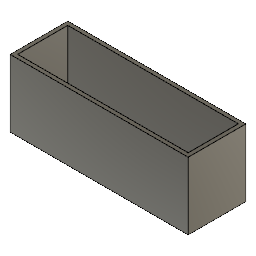
First Test Fit v8 (Autodesk Fusion 360 archive; units mm, degrees)
design "nerf based hopper housing bottom"
Autodesk Fusion 360 part; units mm, degrees
box "BoxPrimitive1" add length 76.2 width 234.95 height 88.9 placed x (0, -1, 0) y (1, 0, 0) z (0, 0, 1) at (0, 0, 0)
shell "Shell1" thickness 5.08 removed faces 1 at (78.3167, -25.4, 88.9)
sketch "flywheel axle" plane through (5.08, 0, 0) normal (1, 0, 0) x (0, 1, 0)
  line L0 (-5.08, 5.08) -> (-5.08, 88.9)
  line L1 (-5.08, 88.9) -> (-71.12, 88.9)
  line L2 (-71.12, 88.9) -> (-71.12, 5.08)
  line L3 (-71.12, 5.08) -> (-5.08, 5.08)
  line L4 (-38.1, 88.9) -> (-38.1, 5.08) construction
  line L5 (-71.12, 46.99) -> (-5.08, 46.99) construction
  circle A0 centre (-38.1, 46.99) radius 3.1
  point P0 (-38.1, 46.99)
  dimension "d10" = 6.2
  constraint midpoint L1 L4.start
  constraint midpoint L3 L4.end
  constraint midpoint L2 L5.start
  constraint midpoint L0 L5.end
  constraint midpoint L4 P0
  constraint coincident P0 A0.centre
  measures "d10" diameter of A0
extrude "Extrude1" add sketch "flywheel axle" along normal blind 228.6 contours A0
sketch "tube slot" plane through (0, 0, 0) normal (0, 1, 0) x (-1, 0, 0)
  line L0 (-234.95, 88.9) -> (-234.95, 0)
  line L1 (-234.95, 0) -> (0, 0)
  line L2 (0, 0) -> (0, 88.9)
  line L3 (0, 88.9) -> (-234.95, 88.9)
  line L4 (-233.68, 11.3178) -> (-1.905, 11.3178)
  line L5 (-1.905, 11.3178) -> (-1.905, 5.08)
  line L6 (-1.905, 5.08) -> (-233.68, 5.08)
  line L7 (-233.68, 5.08) -> (-233.68, 11.3178)
  dimension "d11" = 231.775
  dimension "d13" = 6.2378
  dimension "d14" = 1.27
  dimension "d15" = 5.08
  constraint horizontal L4
  constraint vertical L5
  constraint horizontal L6
  constraint vertical L7
  measures "d11" distance of L4.start L4.end
  measures "d13" distance of L4.end L5.end
  measures "d14" distance of L0 L7
  measures "d15" distance of L1 L6
extrude "Extrude2" cut sketch "tube slot" against normal blind 12.7 contours L4 L5 L6 L7
named bodies: "bottom hopper"

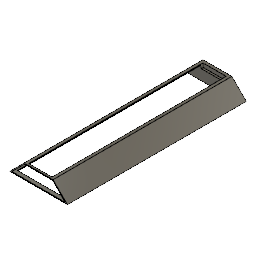
design "nerf based hopper housing V2"
Autodesk Fusion 360 part; units mm, degrees
sketch "top hopper side" plane through (0, 0, 0) normal (0, 1, 0) x (1, 0, 0)
  line L0 (-76.2, 0) -> (0, 0)
  line L1 (0, 0) -> (-19.05, -19.05)
  line L2 (-19.05, -19.05) -> (-57.15, -19.05)
  line L3 (-57.15, -19.05) -> (-76.2, 0)
  dimension "d12" = 76.2
  dimension "d13" = 38.1
  dimension "d14" = 45
  constraint horizontal L0
  constraint parallel L0 L2
  constraint perpendicular L1 L3
  constraint coincident L0.end L1.start
  measures "d12" distance of L0.start L0.end
  measures "d13" distance of L1.end L2.end
  measures "d14" angle of L0 L1
extrude "Extrude3" add sketch "top hopper side" along normal blind 234.95
sketch "side cutout" plane through (0, 0, 0) normal (0, -1, 0) x (1, 0, 0)
  line L0 (-19.05, 19.05) -> (-57.15, 19.05)
  line L1 (-57.15, 19.05) -> (-76.2, 0)
  line L2 (-76.2, 0) -> (0, 0)
  line L3 (0, 0) -> (-19.05, 19.05)
  line L4 (-76.2, 0) -> (-57.15, 19.05)
  line L5 (-19.05, 19.05) -> (0, 0)
  line L6 (-76.2, 0) -> (0, 0)
  line L7 (-57.15, 19.05) -> (-19.05, 19.05)
  line L8 (-73.1339, 1.27) -> (-3.0661, 1.27)
  line L9 (-19.5761, 17.78) -> (-3.0661, 1.27)
  line L10 (-56.6239, 17.78) -> (-19.5761, 17.78)
  line L11 (-73.1339, 1.27) -> (-56.6239, 17.78)
  dimension "d17" = 1.27
  constraint coincident L1.end L2.start
  constraint coincident L0.end L1.start
  constraint coincident L0.start L3.end
  constraint coincident L2.end L3.start
extrude "Extrude4" cut sketch "side cutout" against normal blind 228.6 contours L8 L9 L10 L11
sketch "bottom cutout" plane through (0, 0, 0) normal (0, 0, -1) x (1, 0, 0)
  line L0 (0, 0) -> (-76.2, 0)
  line L1 (-76.2, 0) -> (-76.2, -234.95)
  line L2 (-76.2, -234.95) -> (0, -234.95)
  line L3 (0, -234.95) -> (0, 0)
  line L4 (-5.08, -5.08) -> (-70.7474, -5.08)
  line L5 (-70.7474, -5.08) -> (-70.7474, -228.6)
  line L6 (-5.08, -228.6) -> (-5.08, -5.08)
  line L7 (-5.08, -228.6) -> (-70.7474, -228.6)
  dimension "d20" = 223.52
  dimension "d21" = 65.6674
  dimension "d22" = 5.08
  dimension "d23" = 5.08
  constraint horizontal L4
  constraint vertical L5
  constraint vertical L6
  constraint perpendicular L5 L7
  measures "d20" distance of L4.start L6.start
  measures "d21" distance of L5.end L6.start
  measures "d22" distance of L3 L6
  measures "d23" distance of L0 L4
extrude "Extrude5" cut sketch "bottom cutout" against normal blind 2.54 contours L4 L5 L6 L7
sketch "top cutout" plane through (0, 0, 19.05) normal (0, 0, 1) x (-1, 0, 0)
  line L0 (57.15, 0) -> (19.05, 0)
  line L1 (19.05, 0) -> (19.05, -234.95)
  line L2 (19.05, -234.95) -> (57.15, -234.95)
  line L3 (57.15, -234.95) -> (57.15, 0)
  line L4 (53.34, -2.54) -> (22.86, -2.54)
  line L5 (22.86, -2.54) -> (22.86, -231.14)
  line L6 (22.86, -231.14) -> (53.34, -231.14)
  line L7 (53.34, -231.14) -> (53.34, -2.54)
  dimension "d26" = 228.6
  dimension "d27" = 30.48
  dimension "d28" = 3.81
  dimension "d29" = 2.54
  constraint horizontal L4
  constraint vertical L5
  constraint horizontal L6
  constraint vertical L7
  measures "d26" distance of L4.start L6.end
  measures "d27" distance of L5.end L6.end
  measures "d28" distance of L3 L7
  measures "d29" distance of L0 L4
extrude "Extrude6" cut sketch "top cutout" against normal blind 5.08 contours L4 L5 L6 L7
named bodies: "top hopper"

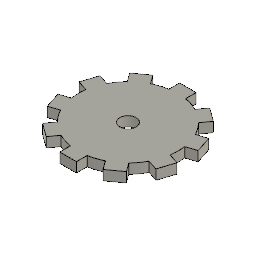
design "Flywheel idea"
Autodesk Fusion 360 part; units mm, degrees
sketch "wheel" plane through (0, 0, 0) normal (0, 0, 1) x (1, 0, 0)
  circle A0 centre (0, 0) radius 19.05
  line L0 (-3.1964, 18.7799) -> (-3.1964, 22.86)
  line L1 (-3.1964, 22.86) -> (3.1964, 22.86)
  line L2 (3.1964, 22.86) -> (3.1964, 18.7799)
  line L3 (-13.6245, 13.3144) -> (-16.0227, 16.6153)
  line L4 (-16.0227, 16.6153) -> (-10.8508, 20.3729)
  line L5 (-10.8508, 20.3729) -> (-8.4526, 17.0721)
  line L6 (-18.8485, 2.7633) -> (-22.7289, 4.0241)
  line L7 (-22.7289, 4.0241) -> (-20.7534, 10.1041)
  line L8 (-20.7534, 10.1041) -> (-16.873, 8.8433)
  line L9 (-16.873, -8.8433) -> (-20.7534, -10.1041)
  line L10 (-20.7534, -10.1041) -> (-22.7289, -4.0241)
  line L11 (-22.7289, -4.0241) -> (-18.8485, -2.7633)
  line L12 (-8.4526, -17.0721) -> (-10.8508, -20.373)
  line L13 (-10.8508, -20.373) -> (-16.0227, -16.6153)
  line L14 (-16.0227, -16.6153) -> (-13.6245, -13.3145)
  line L15 (3.1964, -18.7799) -> (3.1964, -22.86)
  line L16 (3.1964, -22.86) -> (-3.1964, -22.86)
  line L17 (-3.1964, -22.86) -> (-3.1964, -18.7799)
  line L18 (13.6245, -13.3144) -> (16.0227, -16.6153)
  line L19 (16.0227, -16.6153) -> (10.8508, -20.3729)
  line L20 (10.8508, -20.3729) -> (8.4526, -17.0721)
  line L21 (18.8485, -2.7633) -> (22.7289, -4.0241)
  line L22 (22.7289, -4.0241) -> (20.7534, -10.1041)
  line L23 (20.7534, -10.1041) -> (16.873, -8.8433)
  line L24 (16.873, 8.8433) -> (20.7534, 10.1041)
  line L25 (20.7534, 10.1041) -> (22.7289, 4.0241)
  line L26 (22.7289, 4.0241) -> (18.8485, 2.7633)
  line L27 (8.4526, 17.0721) -> (10.8508, 20.373)
  line L28 (10.8508, 20.373) -> (16.0227, 16.6153)
  line L29 (16.0227, 16.6153) -> (13.6245, 13.3145)
  dimension "d1" = 38.1
  dimension "d2" = 6.3929
  dimension "d3" = 4.0801
  dimension "d5" = 360
  constraint coincident A0.centre origin
  constraint coincident A0 L0.start
  constraint vertical L0
  constraint perpendicular L0 L1
  constraint coincident A0 L2.end
  constraint perpendicular L1 L2
  constraint equal L0 L2
  measures "d1" diameter of A0
  measures "d2" distance of L0.end L1.end
  measures "d3" distance of L1.end L2.end
extrude "Extrude1" add sketch "wheel" along normal blind 3.81
sketch "hole punch" plane through (0, 0, 3.81) normal (0, 0, 1) x (-1, 0, 0)
  arc A0 (-8.4526, -17.0721) -> (-3.1964, -18.7799) centre (0, 0) ccw
  line L0 (-3.1964, -18.7799) -> (-3.1964, -22.86)
  line L1 (-3.1964, -22.86) -> (3.1964, -22.86)
  line L2 (3.1964, -22.86) -> (3.1964, -18.7799)
  arc A1 (3.1964, -18.7799) -> (8.4526, -17.0721) centre (0, 0) ccw
  line L3 (8.4526, -17.0721) -> (10.8508, -20.3729)
  line L4 (10.8508, -20.3729) -> (16.0227, -16.6153)
  line L5 (16.0227, -16.6153) -> (13.6245, -13.3144)
  arc A2 (13.6245, -13.3144) -> (16.873, -8.8433) centre (0, 0) ccw
  line L6 (16.873, -8.8433) -> (20.7534, -10.1041)
  line L7 (20.7534, -10.1041) -> (22.7289, -4.0241)
  line L8 (22.7289, -4.0241) -> (18.8485, -2.7633)
  arc A3 (18.8485, -2.7633) -> (18.8485, 2.7633) centre (0, 0) ccw
  line L9 (18.8485, 2.7633) -> (22.7289, 4.0241)
  line L10 (22.7289, 4.0241) -> (20.7534, 10.1041)
  line L11 (20.7534, 10.1041) -> (16.873, 8.8433)
  arc A4 (16.873, 8.8433) -> (13.6245, 13.3145) centre (0, 0) ccw
  line L12 (13.6245, 13.3145) -> (16.0227, 16.6153)
  line L13 (16.0227, 16.6153) -> (10.8508, 20.373)
  line L14 (10.8508, 20.373) -> (8.4526, 17.0721)
  arc A5 (8.4526, 17.0721) -> (3.1964, 18.7799) centre (0, 0) ccw
  line L15 (3.1964, 18.7799) -> (3.1964, 22.86)
  line L16 (3.1964, 22.86) -> (-3.1964, 22.86)
  line L17 (-3.1964, 22.86) -> (-3.1964, 18.7799)
  arc A6 (-3.1964, 18.7799) -> (-8.4526, 17.0721) centre (0, 0) ccw
  line L18 (-8.4526, 17.0721) -> (-10.8508, 20.3729)
  line L19 (-10.8508, 20.3729) -> (-16.0227, 16.6153)
  line L20 (-16.0227, 16.6153) -> (-13.6245, 13.3144)
  arc A7 (-13.6245, 13.3144) -> (-16.873, 8.8433) centre (0, 0) ccw
  line L21 (-16.873, 8.8433) -> (-20.7534, 10.1041)
  line L22 (-20.7534, 10.1041) -> (-22.7289, 4.0241)
  line L23 (-22.7289, 4.0241) -> (-18.8485, 2.7633)
  arc A8 (-18.8485, 2.7633) -> (-18.8485, -2.7633) centre (0, 0) ccw
  line L24 (-18.8485, -2.7633) -> (-22.7289, -4.0241)
  line L25 (-22.7289, -4.0241) -> (-20.7534, -10.1041)
  line L26 (-20.7534, -10.1041) -> (-16.873, -8.8433)
  arc A9 (-16.873, -8.8433) -> (-13.6245, -13.3145) centre (0, 0) ccw
  line L27 (-13.6245, -13.3145) -> (-16.0227, -16.6153)
  line L28 (-16.0227, -16.6153) -> (-10.8508, -20.373)
  line L29 (-10.8508, -20.373) -> (-8.4526, -17.0721)
  circle A10 centre (0, 0) radius 19.05
  line L30 (0.0528, -19.0499) -> (0.0528, 19.0499)
  line L31 (19.05, 0) -> (-19.05, 0)
  constraint coincident A0.centre A1.centre
  constraint coincident A10 L30.start
  constraint coincident A10 L30.end
  constraint vertical L30
  constraint midpoint A3 L31.start
  constraint midpoint A8 L31.end
hole "Hole1" at (0, 0, 3.81) direction (0, 0, -1) diameter 6.2 depth 6.2 tip angle 118
